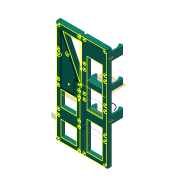
# Autodesk Inventor part: 30_CUBE_openSIM_base
Saved by Autodesk Inventor 2019 (Build 230136000, 136)
## iProperties
Created: 2019-07-01
Part Number: 30_CUBE_openSIM_base
Material: Generic
Document SubType Name: Modeling
Designer: diederichbenedict
Density: 1 g/cm^3
Appearance: IPHT_Türkis
Author: diederichbenedict
Autodesk Inventor part; units mm, degrees
ref_plane "YZ Plane" through (0, 0, 0) normal (1, 0, 0) x (0, 1, 0)
ref_plane "XZ Plane" through (0, 0, 0) normal (0, 1, 0) x (-1, 0, 0)
ref_plane "Work Plane1" through (181.6, 41.8, 16) normal (0, 0, -1) x (-1, 0, 0)
sketch "Sketch1" plane through (0, 41.8, 0) normal (0, 0, 1) x (1, 0, 0)
  circle A0 centre (0.9, -0.9) radius 1.45 construction
  line L0 (4, -1.5) -> (1.5, -4) construction
  line L1 (4, -1.5) -> (4, 4) construction
  line L2 (4, 4) -> (-2, 4) construction
  arc A1 (-2, 4) -> (-4, 2) centre (-2, 2) ccw construction
  line L3 (-4, 2) -> (-4, -4) construction
  line L4 (-4, -4) -> (1.5, -4) construction
  arc A2 (45.8, 2) -> (43.8, 4) centre (43.8, 2) ccw construction
  line L5 (43.8, 4) -> (37.8, 4) construction
  line L6 (37.8, 4) -> (37.8, -1.5) construction
  line L7 (40.3, -4) -> (45.8, -4) construction
  line L8 (45.8, -4) -> (45.8, 2) construction
  circle A3 centre (40.9, -0.9) radius 1.45 construction
  line L9 (37.8, -40.3) -> (40.3, -37.8) construction
  line L10 (37.8, -40.3) -> (37.8, -45.8) construction
  line L11 (37.8, -45.8) -> (43.8, -45.8) construction
  arc A4 (43.8, -45.8) -> (45.8, -43.8) centre (43.8, -43.8) ccw construction
  line L12 (45.8, -43.8) -> (45.8, -37.8) construction
  line L13 (45.8, -37.8) -> (40.3, -37.8) construction
  circle A5 centre (40.9, -40.9) radius 1.45 construction
  circle A6 centre (0.9, -40.9) radius 1.45 construction
  line L14 (1.5, -37.8) -> (4, -40.3) construction
  line L15 (1.5, -37.8) -> (-4, -37.8) construction
  line L16 (-4, -37.8) -> (-4, -43.8) construction
  arc A7 (-4, -43.8) -> (-2, -45.8) centre (-2, -43.8) ccw construction
  line L17 (-2, -45.8) -> (4, -45.8) construction
  line L18 (4, -45.8) -> (4, -40.3) construction
  line L19 (40.3, -4) -> (37.8, -1.5) construction
  line L20 (-2, 154) -> (93.8, 154)
  line L21 (95.8, 152) -> (95.8, -43.8)
  line L22 (93.8, -45.8) -> (-2, -45.8)
  line L23 (-4, -43.8) -> (-4, 152)
  line L24 (90.3, -37.8) -> (90.3, 146)
  line L25 (87.8, 148.5) -> (4, 148.5)
  line L26 (1.5, 146) -> (1.5, -37.8)
  line L27 (4, -40.3) -> (87.8, -40.3)
  line L28 (87.8, -40.3) -> (90.3, -37.8)
  line L29 (4, -40.3) -> (1.5, -37.8)
  line L30 (4, 148.5) -> (1.5, 146)
  line L31 (90.3, 146) -> (87.8, 148.5)
  arc A8 (95.8, 152) -> (93.8, 154) centre (93.8, 152) ccw
  arc A9 (93.8, -45.8) -> (95.8, -43.8) centre (93.8, -43.8) ccw
  arc A10 (-4, -43.8) -> (-2, -45.8) centre (-2, -43.8) ccw
  arc A11 (-2, 154) -> (-4, 152) centre (-2, 152) ccw
  circle A12 centre (1, -1) radius 1.4
  circle A13 centre (40.8, -1) radius 1.4
  circle A14 centre (90.8, -40.8) radius 1.4
  circle A15 centre (1, -40.8) radius 1.4
  circle A16 centre (45.9, 104.1) radius 44.4 construction
  line L32 (45.8, -37.8) -> (87.8, -37.8)
  line L33 (87.8, -37.8) -> (87.8, 146)
  line L34 (45.9, 148.5) -> (45.9, -40.3)
  line L35 (87.8, 146) -> (45.9, 146)
  line L36 (77.4, 111.7) -> (64.2, 111.7) construction
  line L37 (64.2, 96.7) -> (77.4, 96.7) construction
  line L38 (77.4, 61.7) -> (64.2, 61.7) construction
  line L39 (64.2, 46.7) -> (77.4, 46.7) construction
  line L40 (45.9, 111.7) -> (87.8, 111.7)
  line L41 (87.8, 111.7) -> (87.8, 96.7)
  line L42 (87.8, 96.7) -> (45.9, 96.7)
  line L43 (45.9, 96.7) -> (45.9, 111.7)
  line L44 (45.9, 61.7) -> (87.8, 61.7)
  line L45 (87.8, 61.7) -> (87.8, 46.7)
  line L46 (87.8, 46.7) -> (45.9, 46.7)
  line L47 (45.9, 46.7) -> (45.9, 61.7)
  point P0 (95.8, -45.8)
  point P1 (95.8, 154)
  point P2 (-4, -45.8)
  point P3 (90.3, -40.3)
  point P4 (90.3, 148.5)
  point P5 (1.5, 148.5)
  point P6 (1.5, -40.3)
  point P7 (40.8, 149)
  point P8 (45.8, -40.8)
  point P9 (45.9, -37.8)
  point P10 (63.2, 61.7)
  dimension "d34" = 99.8
  dimension "d35" = 199.8
  dimension "d36" = 5.5
  dimension "d37" = 2.5
  dimension "d38" = 2.5
  dimension "d39" = 2.5
  dimension "d40" = 2.5
  dimension "d41" = 2.5
  dimension "d42" = 2.5
  dimension "d43" = 2.5
  dimension "d44" = 2.5
  dimension "d45" = 2
  dimension "d46" = 5
  dimension "d47" = 5
  dimension "d48" = 5
  dimension "d49" = 5
  dimension "d50" = 5
  dimension "d51" = 5
  dimension "d52" = 0.5
  dimension "d53" = 5
  dimension "d54" = 5
  dimension "d55" = 2.8
  dimension "d56" = 2.8
  dimension "d57" = 2.8
  dimension "d58" = 2.8
  constraints: 48 end point, 22 point on line, 9 coincident, 9 parallel, 8 centre point, 8 point on circle, 8 tangent, 5 perpendicular, 4 horizontal, 3 equal radius, 3 midpoint, 2 vertical, 1 vertical alignment, 6 other
  measures "d34" distance of point (95.8, -45.8) point (-4, -45.8)
  measures "d35" distance of point (95.8, 154) point (95.8, -45.8)
  measures "d36" distance between parallel lines of L21 L24
  measures "d37" distance of L27.end point (90.3, -40.3)
  measures "d38" distance of L24.start point (90.3, -40.3)
  measures "d39" distance of L27.start point (1.5, -40.3)
  measures "d40" distance of L26.end point (1.5, -40.3)
  measures "d41" distance of L25.end point (1.5, 148.5)
  measures "d42" distance of L26.start point (1.5, 148.5)
  measures "d43" distance of L24.end point (90.3, 148.5)
  measures "d44" distance of L25.start point (90.3, 148.5)
  measures "d45" radius of A8
  measures "d46" distance from line of point (1, -40.8) L23
  measures "d47" distance from line of L22 point (1, -40.8)
  measures "d48" distance from line of L21 point (90.8, -40.8)
  measures "d49" distance from line of L22 point (90.8, -40.8)
  measures "d50" distance from line of L8 point (40.8, 149)
  measures "d51" distance from line of L20 point (40.8, 149)
  measures "d52" distance from line of point (1, -1) L26
  measures "d53" distance from line of L3 point (1, -1)
  measures "d54" distance from line of L2 point (1, -1)
  measures "d55" diameter of A12
  measures "d56" diameter of A13
  measures "d57" diameter of A14
  measures "d58" diameter of A15
extrude "Extrusion1" add sketch "Sketch1" along normal blind 8 contours L20 A8 L21 A9 L22 A10 L23 A11 | L28 L27 L34 L32 L33 L35 L25 L31 L24 | L27 L29 L26 A12 L30 L25 L34 | L34 L44 L33 L46 | L40 L33 L42 L34 | L26 A12 | A13 picked at (1.6831, -0.6911)
fillet "Fillet1" radius 2 8 edges at (45.9, -4, 8) (95.2142, -3.4142, 8) (95.8, 95.9, 8) (95.2142, 195.2142, 8) (45.9, 195.8, 8) (-3.4142, 195.2142, 8) (-4, 95.9, 8) (-3.4142, -3.4142, 8)
sketch "Sketch2" plane through (-2, -4, 0) normal (0, -1, 0) x (1, 0, 0)
  line L0 (43.8, -4.8712) -> (42.35, -4)
  line L1 (2, -4.8712) -> (0.55, -4)
  line L2 (-2, 0) -> (-2, 6) construction
  line L3 (95.8, 8) -> (0, 8) construction
  line L4 (97.8, 0) -> (97.8, 6) construction
  point P0 (2, 0)
  point P1 (3, 3.1)
  point P2 (92.8, 3.1)
  dimension "d59" = 5
  dimension "d60" = 4.9
  dimension "d61" = 5
  dimension "d62" = 4.9
  constraints: 4 end point, 6 other
  measures "d59" distance from line of point (3, 3.1) L2
  measures "d60" distance from line of point (3, 3.1) L3
  measures "d61" distance from line of point (92.8, 3.1) L4
  measures "d62" distance from line of point (92.8, 3.1) L3
hole "Hole1" at (90.8, -4, 3.1) at (1, -4, 3.1) direction (0, 1, 0) diameter 2.9 depth 6.5 tip angle 118
sketch "Sketch4" plane through (0, 41.8, 8) normal (0, 0, 1) x (1, 0, 0)
  circle A0 centre (1, -40.8) radius 1.4 projected
  circle A1 centre (90.8, -40.8) radius 1.4 projected
  circle A2 centre (1, -1) radius 1.4 projected
  line L0 (-2, -45.8) -> (93.8, -45.8) construction
  line L1 (4, -37.8) -> (4, 146) construction
  circle A3 centre (1, -40.8) radius 1.4 construction
  circle A4 centre (1, -40.8) radius 1.4 construction
  circle A5 centre (1, -1) radius 1.4
  circle A6 centre (1, -40.8) radius 1.4
  line L2 (1, -1) -> (41, -1) construction
  line L3 (41, -1) -> (41, -41) construction
  line L4 (41, -41) -> (1, -41) construction
  line L5 (1, -41) -> (1, -1) construction
  circle A7 centre (1, 9.2) radius 1.4 construction
  circle A8 centre (1, 49) radius 1.4
  circle A9 centre (1, 9.2) radius 1.4
  line L6 (1, 49) -> (41, 49) construction
  line L7 (41, 49) -> (41, 9) construction
  line L8 (41, 9) -> (1, 9) construction
  line L9 (1, 9) -> (1, 49) construction
  circle A10 centre (1, 59.2) radius 1.4 construction
  circle A11 centre (1, 99) radius 1.4
  circle A12 centre (1, 59.2) radius 1.4
  line L10 (1, 99) -> (41, 99) construction
  line L11 (41, 99) -> (41, 59) construction
  line L12 (41, 59) -> (1, 59) construction
  line L13 (1, 59) -> (1, 99) construction
  circle A13 centre (1, 109.2) radius 1.4 construction
  circle A14 centre (1, 149) radius 1.4
  circle A15 centre (1, 109.2) radius 1.4
  line L14 (1, 149) -> (41, 149) construction
  line L15 (41, 149) -> (41, 109) construction
  line L16 (41, 109) -> (1, 109) construction
  line L17 (1, 109) -> (1, 149) construction
  circle A16 centre (51, -40.8) radius 1.4 construction
  circle A17 centre (51, -1) radius 1.4
  circle A18 centre (51, -40.8) radius 1.4
  line L18 (51, -1) -> (91, -1) construction
  line L19 (91, -1) -> (91, -41) construction
  line L20 (91, -41) -> (51, -41) construction
  line L21 (51, -41) -> (51, -1) construction
  circle A19 centre (51, 9.2) radius 1.4 construction
  circle A20 centre (51, 49) radius 1.4
  circle A21 centre (51, 9.2) radius 1.4
  line L22 (51, 49) -> (91, 49) construction
  line L23 (91, 49) -> (91, 9) construction
  line L24 (91, 9) -> (51, 9) construction
  line L25 (51, 9) -> (51, 49) construction
  circle A22 centre (51, 59.2) radius 1.4 construction
  circle A23 centre (51, 99) radius 1.4
  circle A24 centre (51, 59.2) radius 1.4
  line L26 (51, 99) -> (91, 99) construction
  line L27 (91, 99) -> (91, 59) construction
  line L28 (91, 59) -> (51, 59) construction
  line L29 (51, 59) -> (51, 99) construction
  circle A25 centre (51, 109.2) radius 1.4 construction
  circle A26 centre (51, 149) radius 1.4
  circle A27 centre (51, 109.2) radius 1.4
  line L30 (51, 149) -> (91, 149) construction
  line L31 (91, 149) -> (91, 109) construction
  line L32 (91, 109) -> (51, 109) construction
  line L33 (51, 109) -> (51, 149) construction
  point P0 (-2, 4.2)
  point P1 (4, 12.2)
  point P2 (-2, 54.2)
  point P3 (4, 62.2)
  point P4 (-2, 104.2)
  point P5 (4, 112.2)
  point P6 (48, -45.8)
  point P7 (54, -37.8)
  point P8 (48, 4.2)
  point P9 (54, 12.2)
  point P10 (48, 54.2)
  point P11 (54, 62.2)
  point P12 (48, 104.2)
  point P13 (54, 112.2)
  dimension "d106" = 40
  dimension "d107" = 40
  dimension "d110" = 50
  dimension "d113" = 50
  constraints: 64 end point, 24 centre point, 24 coincident, 3 concentric, 2 horizontal, 2 parallel, 1 perpendicular, 1 vertical, 140 other
  measures "d106" distance of L3.end L4.end
  measures "d107" distance of L2.end L3.end
  measures "d110" distance of A0.centre point (1, 9.2)
  measures "d113" distance of A0.centre point (51, -40.8)
hole "Hole2" at (1, 40.8, 8) at (1, 1, 8) at (90.8, 1, 8) at (91, 190.8, 8) at (91, 150.8, 8) at (91, 140.8, 8) at (91, 100.8, 8) at (91, 90.8, 8) at (91, 50.8, 8) at (91, 40.8, 8) at (51, 0.8, 8) at (41, 0.8, 8) at (1, 50.8, 8) at (1, 90.8, 8) at (1, 100.8, 8) at (1, 140.8, 8) at (1, 150.8, 8) at (1, 190.8, 8) at (41, 190.8, 8) at (51, 190.8, 8) at (41, 90.8, 8) at (41, 100.8, 8) at (41, 140.8, 8) at (41, 150.8, 8) at (41, 50.8, 8) at (41, 40.8, 8) at (51, 101, 8) at (51, 90.8, 8) at (51, 140.8, 8) at (51, 151, 8) direction (0, 0, -1) diameter 3.2 depth 12 tip angle 118 counterbore diameter 6 counterbore depth 2.5
sketch "Sketch6" plane through (-4, -2, 0) normal (-1, 0, 0) x (0, 0, 1)
  line L0 (0, -2) -> (6, -2) construction
  line L1 (8, 0) -> (8, 195.8) construction
  line L2 (0, 197.8) -> (6, 197.8) construction
  circle A0 centre (3.1, 192.8) radius 1.4 construction
  circle A1 centre (3.1, 3) radius 1.4 construction
  line L3 (3.1, 3) -> (3.1, 43) construction
  line L4 (3.1, 192.8) -> (3.1, 152.8) construction
  circle A2 centre (3.1, 43) radius 1.4 construction
  circle A3 centre (3.1, 152.8) radius 1.4 construction
  point P0 (0, 2)
  dimension "d63" = 2.8
  dimension "d64" = 2.8
  dimension "d65" = 4.9
  dimension "d66" = 5
  dimension "d67" = 5
  dimension "d68" = 4.9
  dimension "d97" = 40
  dimension "d98" = 40
  constraints: 4 centre point, 4 end point, 2 coincident
  measures "d63" diameter of A0
  measures "d64" diameter of A1
  measures "d65" distance from line of L4.start L1
  measures "d66" distance from line of L4.start L2
  measures "d67" distance from line of L3.start L0
  measures "d68" distance from line of L1 L3.start
  measures "d97" distance of L3.start L3.end
  measures "d98" distance of L4.start L4.end
hole "Hole3" at (-4, 190.8, 3.1) at (-4, 1, 3.1) at (-4, 41, 3.1) at (-4, 150.8, 3.1) direction (1, 0, 0) diameter 2.8 depth 6.5 tip angle 118
sketch "Sketch7" plane through (95.8, -2, 0) normal (1, 0, 0) x (0, 0, -1)
  circle A0 centre (-3.1, 192.8) radius 1.4 projected
  circle A1 centre (-3.1, 3) radius 1.4 projected
  circle A2 centre (-3.1, 43) radius 1.4 projected
  circle A3 centre (-3.1, 152.8) radius 1.4 projected
  point P0 (0, 2)
  constraints: 1 vertical alignment
hole "Hole4" at (95.8, 190.8, 3.1) at (95.8, 1, 3.1) at (95.8, 41, 3.1) at (95.8, 150.8, 3.1) direction (-1, 0, 0) diameter 2.8 depth 6.5 tip angle 118
sketch "Sketch8" plane through (-2, 195.8, 0) normal (0, 1, 0) x (1, 0, 0)
  circle A0 centre (3, -3.1) radius 1.45 projected
  circle A1 centre (92.8, -3.1) radius 1.45 projected
  point P0 (2, 0)
  point P1 (4.45, -3.1)
  point P2 (4.45, -3.1)
  point P3 (94.25, -3.1)
  point P4 (94.25, -3.1)
hole "Hole5" at (1, 195.8, 3.1) at (90.8, 195.8, 3.1) direction (0, -1, 0) diameter 2.8 depth 6.5 tip angle 118
sketch "Sketch23" plane through (0, 41.8, 0) normal (0, 0, -1) x (-1, 0, 0)
  circle A0 centre (-41, 149) radius 1.6 projected
  circle A1 centre (-1, 109) radius 1.6 projected
  circle A2 centre (-1, 59) radius 1.6 projected
  circle A3 centre (-1, 9) radius 1.6 projected
  circle A4 centre (-51, -41) radius 1.6 projected
  circle A5 centre (-91, 9) radius 1.6 projected
  circle A6 centre (-91, 59) radius 1.6 projected
  circle A7 centre (-91, 109) radius 1.6 projected
  circle A8 centre (-90.8, -40.8) radius 1.6 projected
  circle A9 centre (-1, -1) radius 1.6 projected
  circle A10 centre (-1, -40.8) radius 1.6 projected
  circle A11 centre (-91, 149) radius 1.6 projected
  circle A12 centre (-91, 99) radius 1.6 projected
  circle A13 centre (-91, 49) radius 1.6 projected
  circle A14 centre (-91, -1) radius 1.6 projected
  circle A15 centre (-41, -41) radius 1.6 projected
  circle A16 centre (-1, 49) radius 1.6 projected
  circle A17 centre (-1, 99) radius 1.6 projected
  circle A18 centre (-1, 149) radius 1.6 projected
  circle A19 centre (-51, 149) radius 1.6 projected
  line L0 (-87.8, 111.7) -> (-45.9, 111.7) projected
  line L1 (-87.8, 111.7) -> (-87.8, 146) projected
  line L2 (-87.8, 146) -> (-45.9, 146) projected
  line L3 (-45.9, 146) -> (-45.9, 111.7) projected
  line L4 (-45.9, 96.7) -> (-45.9, 61.7) projected
  line L5 (-87.8, 61.7) -> (-45.9, 61.7) projected
  line L6 (-87.8, 61.7) -> (-87.8, 96.7) projected
  line L7 (-45.9, 96.7) -> (-87.8, 96.7) projected
  line L8 (-45.9, -37.8) -> (-87.8, -37.8) projected
  line L9 (-87.8, -37.8) -> (-87.8, 46.7) projected
  line L10 (-45.9, 46.7) -> (-87.8, 46.7) projected
  line L11 (-45.9, 46.7) -> (-45.9, -37.8) projected
  line L12 (-95.8, 152) -> (-95.8, -43.8) projected
  arc A20 (-95.8, -43.8) -> (-93.8, -45.8) centre (-93.8, -43.8) ccw projected
  line L13 (-93.8, -45.8) -> (2, -45.8) projected
  arc A21 (2, -45.8) -> (4, -43.8) centre (2, -43.8) ccw projected
  line L14 (4, -43.8) -> (4, 152) projected
  arc A22 (4, 152) -> (2, 154) centre (2, 152) ccw projected
  line L15 (2, 154) -> (-93.8, 154) projected
  arc A23 (-93.8, 154) -> (-95.8, 152) centre (-93.8, 152) ccw projected
  point P0 (0, -41.8)
extrude "Extrusion15" add sketch "Sketch23" against normal up to surface (8 mm away) contours L1 L2 L3 L0 | L4 L5 L6 L7 | L8 L9 L10 L11
sketch "Sketch24" plane through (0, 41.8, 0) normal (0, 0, -1) x (-1, 0, 0)
  circle A0 centre (-40.518, 42.9814) radius 2.6133
  circle A1 centre (-21.1677, 59.6723) radius 2.5
  circle A2 centre (-39.7243, 68.5233) radius 2.5
  point P0 (0, -41.8)
  constraints: 3 centre point, 6 other
hole "Hole7" at (40.518, 84.7814, 0) at (39.7243, 110.3233, 0) at (21.1677, 101.4723, 0) direction (0, 0, 1) diameter 2.8 depth 8 tip angle 118 counterbore diameter 7 counterbore depth 2
sketch "Sketch25" plane through (0, 41.8, 0) normal (0, 0, -1) x (-1, 0, 0)
  circle A0 centre (-18.2427, 108.6137) radius 1.4
  circle A1 centre (-3.5305, 101.5964) radius 1.4
  line L0 (-34.9278, 89.4278) -> (-14.1642, 132.9595) construction
  line L1 (-7.9405, 76.5555) -> (12.8231, 120.0872) construction
  line L2 (-34.9278, 89.4278) -> (-14.1642, 132.9595)
  line L3 (-14.1642, 132.9595) -> (12.8231, 120.0872)
  line L4 (12.8231, 120.0872) -> (-7.9405, 76.5555)
  line L5 (-7.9405, 76.5555) -> (-34.9278, 89.4278)
  line L6 (4, -43.8) -> (4, 152) projected
  line L7 (4, 124.2956) -> (4, 101.5892)
  point P0 (0, -41.8)
  constraints: 14 end point, 4 point on line, 2 centre point, 2 parallel, 1 perpendicular, 10 other
ref_plane "Work Plane5" through (-11.0179, 119.2166, -1.971) normal (0, 0, 1) x (0.9025853, 0.4305111, 0)
extrude "Extrusion16" add sketch "Sketch25" along normal up to surface (1.971 mm away) contours L2 L3 L6 L4 L5
sketch "Sketch26" plane through (0, 41.8, 8) normal (0, 0, 1) x (1, 0, 0)
  arc A0 (4.2248, 102.8121) -> (4.9122, 101.3708) centre (3.5305, 101.5964) ccw
  arc A1 (17.5484, 107.3979) -> (16.8609, 108.8393) centre (18.2427, 108.6137) ccw
  circle A2 centre (3.5305, 101.5964) radius 1.5
  circle A3 centre (18.2427, 108.6137) radius 1.4 projected
  circle A4 centre (18.2427, 108.6137) radius 1.5
  point P0 (0, -41.8)
  dimension "d170" = 3
  dimension "d171" = 3
  constraints: 4 centre point, 4 point on circle, 2 coincident, 8 other
  measures "d170" diameter of A2
  measures "d171" diameter of A4
hole "Hole8" at (3.5305, 143.3964, 8) at (18.2427, 150.4137, 8) direction (0, 0, -1) diameter 3.3 depth 8 tip angle 118 counterbore diameter 7 counterbore depth 4
ref_plane "Work Plane6" through (-2, 180.8, 0) normal (0, 1, 0) x (1, 0, 0)
sketch "Sketch27" plane through (-2, 180.8, 0) normal (0, 1, 0) x (1, 0, 0)
  circle A0 centre (72.821, 16.921) radius 15.24 construction
  circle A1 centre (72.821, 16.921) radius 14.99 construction
  line L0 (72.821, 16.921) -> (88.9923, 33.0923) construction
  line L1 (72.821, 16.921) -> (95.6907, 16.921) construction
  arc A2 (62.2214, 6.3214) -> (83.4205, 27.5205) centre (72.821, 16.921) ccw
  arc A3 (58.0587, 14.318) -> (62.2214, 6.3214) centre (72.821, 16.921) ccw
  line L2 (58.0587, 14.318) -> (72.821, 16.921) construction
  line L3 (58.0587, 14.318) -> (55.0587, 14.318) construction
  line L4 (55.0587, 14.318) -> (58.0587, 14.318)
  line L5 (55.0587, 14.318) -> (55.0587, 0)
  line L6 (0, 0) -> (95.8, 0) projected
  line L7 (83.4205, 27.5205) -> (83.4205, 30.5205)
  line L8 (83.4205, 30.5205) -> (90.5546, 30.5205)
  line L9 (90.5546, 30.5205) -> (90.5546, 0)
  point P0 (2, 0)
  dimension "d180" = 0.25
  dimension "d181" = 45
  dimension "d182" = 145
  dimension "d183" = 3
  dimension "d184" = 3
  constraints: 18 end point, 7 point on circle, 4 centre point, 4 point on line, 3 perpendicular, 2 concentric, 2 horizontal, 1 equal length, 1 parallel, 2 other
  measures "d180" radial gap between concentric circles of A0 A1
  measures "d181" angle of L1 L0
  measures "d182" angle of L0 L2
  measures "d183" distance of L2.start L3.end
  measures "d184" distance of L7.start L7.end
extrude "Extrusion17" add sketch "Sketch27" against normal blind 15
fillet "Fillet2" radius 2 7 edges at (53.0587, 173.3, -14.318) (56.0587, 173.3, -14.318) (81.4205, 173.3, -30.5205) (88.5546, 173.3, -30.5205) (53.0587, 173.3, 0) (88.5546, 173.3, 0) (81.4205, 173.3, -27.5205)
ref_plane "Work Plane7" through (-2, 75.8, 0) normal (0, 1, 0) x (1, 0, 0)
sketch "Sketch28" plane through (-2, 75.8, 0) normal (0, 1, 0) x (1, 0, 0)
  arc A0 (83.4205, 28.3188) -> (83.9373, 26.9771) centre (85.4205, 28.3188) ccw projected
  arc A1 (58.9142, 11.3262) -> (83.9373, 26.9771) centre (72.821, 16.921) ccw projected
  arc A2 (58.9142, 11.3262) -> (55.0587, 10.5797) centre (57.0587, 10.5797) ccw projected
  line L0 (55.0587, 2) -> (55.0587, 10.5797) projected
  arc A3 (53.0587, 0) -> (55.0587, 2) centre (53.0587, 2) ccw projected
  line L1 (92.5546, 0) -> (53.0587, 0) projected
  arc A4 (90.5546, 2) -> (92.5546, 0) centre (92.5546, 2) ccw projected
  line L2 (90.5546, 28.5205) -> (90.5546, 2) projected
  arc A5 (90.5546, 28.5205) -> (88.5546, 30.5205) centre (88.5546, 28.5205) ccw projected
  line L3 (85.4205, 30.5205) -> (88.5546, 30.5205) projected
  arc A6 (85.4205, 30.5205) -> (83.4205, 28.5205) centre (85.4205, 28.5205) ccw projected
  line L4 (83.4205, 28.3188) -> (83.4205, 28.5205) projected
  point P0 (2, 0)
extrude "Extrusion18" add sketch "Sketch28" against normal blind 15
sketch "Sketch29" plane through (0, 41.8, 8) normal (0, 0, 1) x (1, 0, 0)
  point P0 (0, -41.8)
sketch "Sketch30" plane through (0, 41.8, 0) normal (0, 0, -1) x (-1, 0, 0)
  line L0 (-90.5546, 19) -> (-90.5546, 34) projected
  line L1 (-90.5546, 34) -> (-51.0587, 34) projected
  line L2 (-51.0587, 19) -> (-51.0587, 34) projected
  line L3 (-51.0587, 19) -> (-90.5546, 19) projected
  line L4 (-90.5546, 139) -> (-51.0587, 139) projected
  line L5 (-51.0587, 124) -> (-51.0587, 139) projected
  line L6 (-51.0587, 124) -> (-90.5546, 124) projected
  circle A0 centre (-91, 109) radius 1.6 projected
  line L7 (-90.5546, 139) -> (-90.5546, 124) projected
  line L8 (-14.1642, 132.9595) -> (4, 124.2956) projected
  arc A1 (4, 152) -> (2, 154) centre (2, 152) ccw projected
  line L9 (2, 154) -> (-93.8, 154) projected
  arc A2 (-93.8, 154) -> (-95.8, 152) centre (-93.8, 152) ccw projected
  line L10 (-95.8, 152) -> (-95.8, -43.8) projected
  arc A3 (-95.8, -43.8) -> (-93.8, -45.8) centre (-93.8, -43.8) ccw projected
  line L11 (-93.8, -45.8) -> (2, -45.8) projected
  arc A4 (2, -45.8) -> (4, -43.8) centre (2, -43.8) ccw projected
  line L12 (4, 101.5892) -> (-7.9405, 76.5555) projected
  line L13 (-7.9405, 76.5555) -> (-34.9278, 89.4278) projected
  line L14 (-34.9278, 89.4278) -> (-14.1642, 132.9595) projected
  circle A5 centre (-39.7243, 68.5233) radius 3.5 projected
  circle A6 centre (-40.518, 42.9814) radius 3.5 projected
  circle A7 centre (-21.1677, 59.6723) radius 3.5 projected
  circle A8 centre (-41, 149) radius 1.6 projected
  circle A9 centre (-1, 59) radius 1.6 projected
  circle A10 centre (-1, 9) radius 1.6 projected
  circle A11 centre (-51, -41) radius 1.6 projected
  circle A12 centre (-91, 9) radius 1.6 projected
  circle A13 centre (-91, 59) radius 1.6 projected
  circle A14 centre (-90.8, -40.8) radius 1.6 projected
  circle A15 centre (-1, -1) radius 1.6 projected
  circle A16 centre (-1, -40.8) radius 1.6 projected
  circle A17 centre (-91, 149) radius 1.6 projected
  circle A18 centre (-91, 99) radius 1.6 projected
  circle A19 centre (-91, 49) radius 1.6 projected
  circle A20 centre (-91, -1) radius 1.6 projected
  circle A21 centre (-41, -41) radius 1.6 projected
  circle A22 centre (-1, 49) radius 1.6 projected
  circle A23 centre (-1, 149) radius 1.6 projected
  circle A24 centre (-51, 149) radius 1.6 projected
  line L15 (4, -45.8) -> (-45.8, -45.8) construction
  line L16 (-45.8, -45.8) -> (-45.8, 4) construction
  line L17 (-45.8, 4) -> (4, 4) construction
  line L18 (4, 4) -> (4, -45.8) construction
  line L19 (-95.8, -45.8) -> (-46, -45.8) construction
  line L20 (-46, -45.8) -> (-46, 4) construction
  line L21 (-46, 4) -> (-95.8, 4) construction
  line L22 (-95.8, 4) -> (-95.8, -45.8) construction
  line L23 (-56.9142, 124) -> (-85.811, 124) construction
  line L24 (-81.9373, 124) -> (-81.9373, 139) construction
  line L25 (-56.9142, 124) -> (-81.9373, 124) construction
  line L26 (-56.9142, 139) -> (-56.9142, 124) construction
  line L27 (-56.9142, 139) -> (-81.9373, 139) construction
  circle A25 centre (-70.8, -21) radius 25 construction
  line L28 (-35.9, -36) -> (-5.9, -36) construction
  line L29 (-5.9, -36) -> (-5.9, -6) construction
  line L30 (-5.9, -6) -> (-35.9, -6) construction
  line L31 (-35.9, -6) -> (-35.9, -36) construction
  line L32 (-35.9, -36) -> (-5.9, -6) construction
  line L33 (-5.9, -36) -> (-35.9, -6) construction
  line L34 (-35.9, -6) -> (-5.9, -6)
  line L35 (-5.9, -6) -> (-5.9, -36)
  line L36 (-5.9, -36) -> (-35.9, -36)
  line L37 (-35.9, -36) -> (-35.9, -6)
  line L38 (-35.9, -6) -> (-5.9, -36) construction
  line L39 (-5.9, -6) -> (-35.9, -36) construction
  line L40 (4, 4) -> (-45.8, 4)
  line L41 (-45.8, 4) -> (-45.8, 53.8)
  line L42 (-45.8, 53.8) -> (4, 53.8)
  line L43 (4, 53.8) -> (4, 4) construction
  circle A26 centre (-20.9, 28.9) radius 24.9
  line L44 (-5.9, 43.9) -> (-35.9, 43.9)
  line L45 (-35.9, 43.9) -> (-35.9, 13.9)
  line L46 (-35.9, 13.9) -> (-5.9, 13.9)
  line L47 (-5.9, 13.9) -> (-5.9, 43.9)
  line L48 (-5.9, 43.9) -> (-35.9, 13.9) construction
  line L49 (-35.9, 43.9) -> (-5.9, 13.9) construction
  line L50 (-55.8, -36) -> (-85.8, -36)
  line L51 (-85.8, -36) -> (-85.8, 9)
  line L52 (-85.8, 9) -> (-55.8, 9)
  line L53 (-55.8, 9) -> (-55.8, -36)
  line L54 (4, 124.2956) -> (4, 152) projected
  line L55 (4, -43.8) -> (4, 101.5892) projected
  line L56 (-45.8, 66.6337) -> (-9.6212, 142.4842)
  line L57 (-7.9405, 76.5555) -> (-34.9278, 89.4278) projected
  line L58 (-9.6212, 142.4842) -> (-45.8, 142.4842)
  line L59 (-45.8, 142.4842) -> (-45.8, 66.6337)
  line L60 (-90.5546, 34) -> (-51.0587, 34) projected
  line L61 (-55.8, 124) -> (-85.8, 124)
  line L62 (-85.8, 124) -> (-85.8, 34)
  line L63 (-85.8, 34) -> (-55.8, 34)
  line L64 (-55.8, 34) -> (-55.8, 124)
  line L65 (-51.0587, 19) -> (-90.5546, 19) projected
  line L66 (-55.8, 9) -> (-85.8, 9)
  line L67 (-85.8, 9) -> (-85.8, 19)
  line L68 (-85.8, 19) -> (-55.8, 19)
  line L69 (-55.8, 19) -> (-55.8, 9)
  circle A27 centre (-51, 109.2) radius 1.6 projected
  point P0 (0, -41.8)
  point P1 (-20.9, -21)
  point P2 (-20.9, -21)
  dimension "d191" = 49.8
  dimension "d192" = 49.8
  dimension "d193" = 49.8
  dimension "d194" = 49.8
  dimension "d196" = 30
  dimension "d197" = 30
  dimension "d198" = 49.8
  dimension "d199" = 30
  dimension "d200" = 30
  dimension "d205" = 45
  constraints: 90 end point, 18 parallel, 11 perpendicular, 10 horizontal, 7 midpoint, 6 tangent, 5 point on line, 2 centre point
  measures "d191" distance of L16.end L17.end
  measures "d192" distance of L15.end L16.end
  measures "d193" distance of L21.end L20.end
  measures "d194" distance of L20.end L19.end
  measures "d196" distance of L30.end L29.end
  measures "d197" distance of L29.end L28.end
  measures "d198" distance of L40.end L41.end
  measures "d199" distance of L46.end L45.end
  measures "d200" distance of L45.end L44.end
  measures "d205" distance of L50.end L51.end
extrude "Extrusion19" cut sketch "Sketch30" against normal blind 15 contours L3 L69 L52 L67 | L62 L6 L64 L1 | L52 L53 L50 L51 | L14 L56 L59 L58 | L34 L35 L36 L37 | L47 L46 L45 L44
sketch "Sketch31" plane through (-2, 180.8, 0) normal (0, 1, 0) x (1, 0, 0)
  circle A0 centre (47.8, -1.2) radius 3.1
  line L0 (97.8, -1.7) -> (97.8, -4.5) projected
  line L1 (95.8, 0) -> (0, 0) projected
  point P0 (2, 0)
  dimension "d207" = 6.2
  dimension "d208" = 50
  dimension "d209" = 1.2
  constraints: 1 centre point
  measures "d207" diameter of A0
  measures "d208" distance from line of A0.centre L0
  measures "d209" distance from line of A0.centre L1
extrude "Extrusion20" cut sketch "Sketch31" along normal through all both and the other way through all
sketch "Sketch34" plane through (0, 41.8, 8) normal (0, 0, 1) x (1, 0, 0)
  line L0 (85.8, 124) -> (85.8, 34) projected
  line L1 (85.8, 34) -> (55.8, 34) projected
  line L2 (85.8, -36) -> (55.8, -36) projected
  line L3 (55.8, -36) -> (55.8, 19) projected
  line L4 (55.8, 19) -> (85.8, 19) projected
  line L5 (85.8, 19) -> (85.8, -36) projected
  line L6 (5.9, -6) -> (35.9, -6) projected
  line L7 (35.9, -6) -> (35.9, -36) projected
  line L8 (35.9, -36) -> (5.9, -36) projected
  line L9 (5.9, -36) -> (5.9, -6) projected
  line L10 (9.6212, 142.4842) -> (45.8, 142.4842) projected
  line L11 (45.8, 142.4842) -> (45.8, 66.6337) projected
  line L12 (45.8, 66.6337) -> (9.6212, 142.4842) projected
  line L13 (35.9, 43.9) -> (35.9, 13.9) projected
  line L14 (35.9, 13.9) -> (5.9, 13.9) projected
  line L15 (5.9, 13.9) -> (5.9, 43.9) projected
  line L16 (5.9, 43.9) -> (35.9, 43.9) projected
  arc A0 (3.8657, 98.1124) -> (0.0391, 101.842) centre (3.5305, 101.5964) ccw projected
  arc A1 (-2, 99) -> (3.8657, 98.1124) centre (1, 99) ccw projected
  line L17 (-2, 59) -> (-2, 99) projected
  circle A2 centre (1, 59) radius 3 projected
  line L18 (-2, 49) -> (-2, 59) projected
  circle A3 centre (1, 49) radius 3 projected
  line L19 (-2, 9) -> (-2, 49) projected
  circle A4 centre (1, 9) radius 3 projected
  line L20 (-2, -1) -> (-2, 9) projected
  circle A5 centre (1, -1) radius 3 projected
  line L21 (-2, -40.8) -> (-2, -1) projected
  arc A6 (1, -43.8) -> (-2, -40.8) centre (1, -40.8) ccw projected
  line L22 (39.923, -43.8) -> (1, -43.8) projected
  arc A7 (42.077, -43.8) -> (39.923, -43.8) centre (41, -41) ccw projected
  line L23 (49.923, -43.8) -> (42.077, -43.8) projected
  arc A8 (52.077, -43.8) -> (49.923, -43.8) centre (51, -41) ccw projected
  line L24 (90.8, -43.8) -> (52.077, -43.8) projected
  arc A9 (93.8, -40.8) -> (90.8, -43.8) centre (90.8, -40.8) ccw projected
  line L25 (93.8, -2.077) -> (93.8, -40.8) projected
  arc A10 (93.8, 0.077) -> (93.8, -2.077) centre (91, -1) ccw projected
  line L26 (93.8, 7.923) -> (93.8, 0.077) projected
  arc A11 (93.8, 10.077) -> (93.8, 7.923) centre (91, 9) ccw projected
  line L27 (93.8, 47.923) -> (93.8, 10.077) projected
  arc A12 (93.8, 50.077) -> (93.8, 47.923) centre (91, 49) ccw projected
  line L28 (93.8, 57.923) -> (93.8, 50.077) projected
  arc A13 (93.8, 60.077) -> (93.8, 57.923) centre (91, 59) ccw projected
  line L29 (93.8, 97.923) -> (93.8, 60.077) projected
  arc A14 (93.8, 100.077) -> (93.8, 97.923) centre (91, 99) ccw projected
  line L30 (93.8, 107.923) -> (93.8, 100.077) projected
  arc A15 (93.8, 110.077) -> (93.8, 107.923) centre (91, 109) ccw projected
  line L31 (93.8, 147.923) -> (93.8, 110.077) projected
  arc A16 (91, 152) -> (93.8, 147.923) centre (91, 149) ccw projected
  line L32 (51, 152) -> (91, 152) projected
  circle A17 centre (51, 149) radius 3 projected
  line L33 (41, 152) -> (51, 152) projected
  circle A18 centre (41, 149) radius 3 projected
  line L34 (1, 152) -> (41, 152) projected
  arc A19 (-2, 149) -> (1, 152) centre (1, 149) ccw projected
  line L35 (-2, 109) -> (-2, 149) projected
  circle A20 centre (1, 109) radius 3 projected
  line L36 (-2, 99) -> (-2, 109) projected
  arc A21 (0.0391, 101.842) -> (-2, 99) centre (1, 99) ccw projected
  circle A22 centre (18.2427, 108.6137) radius 3.5 projected
  circle A23 centre (39.7243, 68.5233) radius 1.4 projected
  circle A24 centre (40.518, 42.9814) radius 1.4 projected
  circle A25 centre (21.1677, 59.6723) radius 1.4 projected
  arc A26 (49.3417, 61.7) -> (52.6583, 61.7) centre (51, 59.2) ccw projected
  line L37 (52.6583, 61.7) -> (49.3417, 61.7) projected
  arc A27 (49.3417, 111.7) -> (52.6583, 111.7) centre (51, 109.2) ccw projected
  line L38 (52.6583, 111.7) -> (49.3417, 111.7) projected
  line L39 (49.0739, 46.7) -> (52.9261, 46.7) projected
  arc A28 (52.9261, 46.7) -> (49.0739, 46.7) centre (51, 49) ccw projected
  circle A29 centre (41, -1) radius 3 projected
  circle A30 centre (41, 59) radius 3 projected
  circle A31 centre (41, 49) radius 3 projected
  circle A32 centre (41, 9) radius 3 projected
  line L40 (49.0739, 96.7) -> (52.9261, 96.7) projected
  arc A33 (52.9261, 96.7) -> (49.0739, 96.7) centre (51, 99) ccw projected
  line L41 (9.6212, 135.0512) -> (38, 72.8149)
  line L42 (38, 72.8149) -> (30.9112, 72.8149)
  line L43 (42.7, -45.8) -> (42.7, 154) projected
  line L44 (30.9112, 72.8149) -> (30.9112, 46.7)
  line L45 (30.9112, 46.7) -> (5.9734, 46.7)
  line L46 (5.9734, 46.7) -> (5.9734, 143.0509)
  line L47 (5.9734, 143.0509) -> (9.6212, 135.0512)
  line L48 (55.8, 34) -> (55.8, 124) projected
  line L49 (55.8, 124) -> (85.8, 124) projected
  point P0 (0, -41.8)
  constraints: 12 end point, 5 horizontal alignment, 4 perpendicular, 2 vertical alignment, 1 collinear, 1 point on line
ref_plane "Work Plane8" through (-2, 115.8, 0) normal (0, 1, 0) x (1, 0, 0)
sketch "Sketch35" plane through (-2, 115.8, 0) normal (0, 1, 0) x (1, 0, 0)
  arc A0 (83.4205, 28.3188) -> (83.9373, 26.9771) centre (85.4205, 28.3188) ccw projected
  arc A1 (58.9142, 11.3262) -> (83.9373, 26.9771) centre (72.821, 16.921) ccw projected
  arc A2 (58.9142, 11.3262) -> (55.0587, 10.5797) centre (57.0587, 10.5797) ccw projected
  line L0 (55.0587, 10.5797) -> (55.0587, 2) projected
  arc A3 (53.0587, 0) -> (55.0587, 2) centre (53.0587, 2) ccw projected
  line L1 (57.8, 0) -> (53.0587, 0) projected
  line L2 (57.8, 0) -> (57.8, -8) projected
  line L3 (87.8, -8) -> (57.8, -8) projected
  line L4 (87.8, 0) -> (87.8, -8) projected
  line L5 (92.5546, 0) -> (87.8, 0) projected
  arc A4 (90.5546, 2) -> (92.5546, 0) centre (92.5546, 2) ccw projected
  line L6 (90.5546, 2) -> (90.5546, 28.5205) projected
  arc A5 (90.5546, 28.5205) -> (88.5546, 30.5205) centre (88.5546, 28.5205) ccw projected
  line L7 (88.5546, 30.5205) -> (85.4205, 30.5205) projected
  arc A6 (85.4205, 30.5205) -> (83.4205, 28.5205) centre (85.4205, 28.5205) ccw projected
  line L8 (83.4205, 28.5205) -> (83.4205, 28.3188) projected
  point P0 (2, 0)
extrude "Extrusion22" add sketch "Sketch35" along normal blind 10
sketch "Sketch36" plane through (0, 41.8, 8) normal (0, 0, 1) x (1, 0, 0)
  line L0 (85.8, 74) -> (85.8, 34) construction
  line L1 (85.8, 34) -> (55.8, 34) construction
  line L2 (55.8, 34) -> (55.8, 74) construction
  line L3 (55.8, 74) -> (85.8, 74) construction
  line L4 (55.8, 84) -> (85.8, 84) construction
  line L5 (55.8, 84) -> (55.8, 124) construction
  line L6 (55.8, 124) -> (85.8, 124) construction
  line L7 (85.8, 124) -> (85.8, 84) construction
  line L8 (85.8, -36) -> (55.8, -36) construction
  line L9 (55.8, -36) -> (55.8, 19) construction
  line L10 (55.8, 19) -> (85.8, 19) construction
  line L11 (85.8, 19) -> (85.8, -36) construction
  line L12 (5.9, -6) -> (35.9, -6) construction
  line L13 (35.9, -6) -> (35.9, -36) construction
  line L14 (35.9, -36) -> (5.9, -36) construction
  line L15 (5.9, -36) -> (5.9, -6) construction
  line L16 (9.6212, 142.4842) -> (45.8, 142.4842) construction
  line L17 (45.8, 142.4842) -> (45.8, 66.6337) construction
  line L18 (45.8, 66.6337) -> (9.6212, 142.4842) construction
  line L19 (35.9, 43.9) -> (35.9, 13.9) construction
  line L20 (35.9, 13.9) -> (5.9, 13.9) construction
  line L21 (5.9, 13.9) -> (5.9, 43.9) construction
  line L22 (5.9, 43.9) -> (35.9, 43.9) construction
  arc A0 (3.8657, 98.1124) -> (0.0391, 101.842) centre (3.5305, 101.5964) ccw construction
  arc A1 (-2, 99) -> (3.8657, 98.1124) centre (1, 99) ccw construction
  line L23 (-2, 59) -> (-2, 99) construction
  circle A2 centre (1, 59) radius 3 construction
  line L24 (-2, 49) -> (-2, 59) construction
  circle A3 centre (1, 49) radius 3 construction
  line L25 (-2, 9) -> (-2, 49) construction
  circle A4 centre (1, 9) radius 3 construction
  line L26 (-2, -1) -> (-2, 9) construction
  circle A5 centre (1, -1) radius 3 construction
  line L27 (-2, -40.8) -> (-2, -1) construction
  arc A6 (1, -43.8) -> (-2, -40.8) centre (1, -40.8) ccw construction
  line L28 (39.923, -43.8) -> (1, -43.8) construction
  arc A7 (42.077, -43.8) -> (39.923, -43.8) centre (41, -41) ccw construction
  line L29 (49.923, -43.8) -> (42.077, -43.8) construction
  arc A8 (52.077, -43.8) -> (49.923, -43.8) centre (51, -41) ccw construction
  line L30 (90.8, -43.8) -> (52.077, -43.8) construction
  arc A9 (93.8, -40.8) -> (90.8, -43.8) centre (90.8, -40.8) ccw construction
  line L31 (93.8, -2.077) -> (93.8, -40.8) construction
  arc A10 (93.8, 0.077) -> (93.8, -2.077) centre (91, -1) ccw construction
  line L32 (93.8, 7.923) -> (93.8, 0.077) construction
  arc A11 (93.8, 10.077) -> (93.8, 7.923) centre (91, 9) ccw construction
  line L33 (93.8, 47.923) -> (93.8, 10.077) construction
  arc A12 (93.8, 50.077) -> (93.8, 47.923) centre (91, 49) ccw construction
  line L34 (93.8, 57.923) -> (93.8, 50.077) construction
  arc A13 (93.8, 60.077) -> (93.8, 57.923) centre (91, 59) ccw construction
  line L35 (93.8, 97.923) -> (93.8, 60.077) construction
  arc A14 (93.8, 100.077) -> (93.8, 97.923) centre (91, 99) ccw construction
  line L36 (93.8, 107.923) -> (93.8, 100.077) construction
  arc A15 (93.8, 110.077) -> (93.8, 107.923) centre (91, 109) ccw construction
  line L37 (93.8, 147.923) -> (93.8, 110.077) construction
  arc A16 (91, 152) -> (93.8, 147.923) centre (91, 149) ccw construction
  line L38 (51, 152) -> (91, 152) construction
  circle A17 centre (51, 149) radius 3 construction
  line L39 (41, 152) -> (51, 152) construction
  circle A18 centre (41, 149) radius 3 construction
  line L40 (1, 152) -> (41, 152) construction
  arc A19 (-2, 149) -> (1, 152) centre (1, 149) ccw construction
  line L41 (-2, 109) -> (-2, 149) construction
  circle A20 centre (1, 109) radius 3 construction
  line L42 (-2, 99) -> (-2, 109) construction
  arc A21 (0.0391, 101.842) -> (-2, 99) centre (1, 99) ccw construction
  circle A22 centre (18.2427, 108.6137) radius 3.5 construction
  circle A23 centre (39.7243, 68.5233) radius 1.4 construction
  circle A24 centre (40.518, 42.9814) radius 1.4 construction
  circle A25 centre (21.1677, 59.6723) radius 1.4 construction
  arc A26 (49.3417, 61.7) -> (52.6583, 61.7) centre (51, 59.2) ccw construction
  line L43 (52.6583, 61.7) -> (49.3417, 61.7) construction
  arc A27 (49.3417, 111.7) -> (52.6583, 111.7) centre (51, 109.2) ccw construction
  line L44 (52.6583, 111.7) -> (49.3417, 111.7) construction
  line L45 (49.0739, 46.7) -> (52.9261, 46.7) construction
  arc A28 (52.9261, 46.7) -> (49.0739, 46.7) centre (51, 49) ccw construction
  circle A29 centre (41, -1) radius 3 construction
  circle A30 centre (41, 59) radius 3 construction
  circle A31 centre (41, 49) radius 3 construction
  circle A32 centre (41, 9) radius 3 construction
  line L46 (49.0739, 96.7) -> (52.9261, 96.7) construction
  arc A33 (52.9261, 96.7) -> (49.0739, 96.7) centre (51, 99) ccw construction
  line L47 (90.8, -40.8) -> (51, -40.8) construction
  line L48 (51, -40.8) -> (51, -1) construction
  line L49 (51, -1) -> (90.8, -1) construction
  line L50 (90.8, -1) -> (90.8, -40.8) construction
  line L51 (91, 9) -> (51, 9) construction
  line L52 (51, 9) -> (51, 49) construction
  line L53 (51, 49) -> (91, 49) construction
  line L54 (91, 49) -> (91, 9) construction
  line L55 (91, 59) -> (51, 59) construction
  line L56 (51, 59) -> (51, 99) construction
  line L57 (51, 99) -> (91, 99) construction
  line L58 (91, 99) -> (91, 59) construction
  point P0 (0, -41.8)
  point P1 (49.923, -2.077)
  point P2 (49.923, 9)
  constraints: 24 end point, 6 parallel, 5 horizontal alignment, 3 horizontal, 3 perpendicular, 2 coincident, 2 vertical alignment
sketch "Sketch37" plane through (0, 41.8, 8) normal (0, 0, 1) x (1, 0, 0)
  point P0 (0, -41.8)
  point P1 (50.9148, -1.0555)
  point P2 (50.9598, 9.0215)
hole "Hole9" at (50.9148, 40.7445, 8) at (50.9598, 50.8215, 8) direction (0, 0, -1) diameter 2.8 depth 12 tip angle 118 counterbore diameter 6 counterbore depth 2.5
sketch "Sketch38" plane through (-2, 75.8, 0) normal (0, 1, 0) x (1, 0, 0)
  arc A0 (84.2577, 17.5746) -> (61.3842, 17.5746) centre (72.821, 16.921) ccw
  ellipse E0 centre (72.821, 16.921) end of major axis (72.516, 16.921) minor radius 0.2753 (72.821, 16.6457) -> (72.821, 17.1962) ccw
  circle A1 centre (72.821, 16.921) radius 0.2753
  arc A2 (72.821, 17.1962) -> (72.821, 16.6457) centre (72.821, 16.921) ccw
  ellipse E1 centre (74.7289, 16.921) end of major axis (74.4239, 16.921) minor radius 0.2753 (74.4284, 16.8738) -> (74.7502, 17.1956) ccw
  point P0 (2, 0)
  constraints: 4 point on circle, 3 centre point, 22 other
equation "\"d38\" = d37"
equation "\"d39\" = d37"
equation "\"d40\" = d39"
equation "\"d41\" = d37"
equation "\"d42\" = d41"
equation "\"d43\" = d37"
equation "\"d44\" = d43"
body "Solid1"
